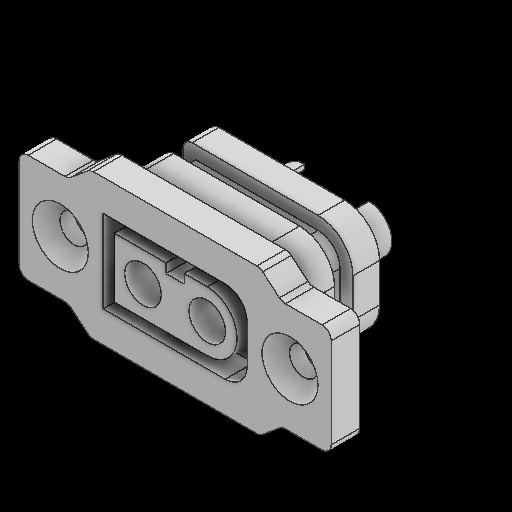
# Autodesk Inventor part: XT60E-F
Saved by Autodesk Inventor 2025.2 (Build 292293000, 293)
## iProperties
Created: 2026-06-05
Part Number: XT60E-F
Material: Generic
Document SubType Name: Modeling
Designer: valer
Density: 1 g/cm^3
Appearance: Default
Author: valer
Autodesk Inventor part; units mm, degrees
ref_plane "YZ Plane" through (0, 0, 0) normal (1, 0, 0) x (0, 1, 0)
ref_plane "XZ Plane" through (0, 0, 0) normal (0, 1, 0) x (-1, 0, 0)
ref_plane "XY Plane" through (0, 0, 0) normal (0, 0, 1) x (1, 0, 0)
sketch "Base" plane through (0, 0, 0) normal (0, 0, 1) x (1, 0, 0)
  line L0 (-17, 5.9) -> (17, 5.9)
  line L1 (17, 5.9) -> (17, -5.9)
  line L2 (17, -5.9) -> (-17, -5.9)
  line L3 (-17, -5.9) -> (-17, 5.9)
  line L4 (-17, 0) -> (17, 0) construction
  line L5 (-9.25, -7.9) -> (9.25, -7.9)
  line L6 (9.25, -7.9) -> (9.25, 7.9)
  line L7 (9.25, 7.9) -> (-9.25, 7.9)
  line L8 (-9.25, 7.9) -> (-9.25, -7.9)
  line L9 (-9.25, -7.9) -> (9.25, 7.9) construction
  line L10 (9.25, -7.9) -> (-9.25, 7.9) construction
  line L11 (-9.25, 7.9) -> (-11.6335, 5.9)
  line L12 (0, 7.9) -> (0, -7.9) construction
  line L13 (9.25, 7.9) -> (11.6335, 5.9)
  line L14 (-9.25, -7.9) -> (-11.6335, -5.9)
  line L15 (9.25, -7.9) -> (11.6335, -5.9)
  circle A0 centre (-12.5, 0) radius 1.55
  circle A1 centre (12.5, 0) radius 1.55
  arc A2 (9.25, 2.1) -> (5.45, 5.9) centre (5.45, 2.1) ccw
  arc A3 (5.45, -5.9) -> (9.25, -2.1) centre (5.45, -2.1) ccw
  circle A4 centre (3.5, 0) radius 2
  circle A5 centre (-3.5, 0) radius 2
  point P0 (0, 0)
  point P1 (0, 0)
  point P2 (0, 0)
  point P3 (5.45, -5.9)
  point P4 (9.25, -2.1)
  point P5 (-9.25, 5.9)
  point P6 (-9.25, -5.9)
  dimension "d0" = 11.8
  dimension "d1" = 15.8
  dimension "d2" = 18.5
  dimension "d3" = 140
  dimension "d4" = 3.1
  dimension "d5" = 3.8
  dimension "d6" = 4
  dimension "d7" = 3.5
  dimension "d8" = 25
  dimension "d9" = 34
  constraints: 32 end point, 8 midpoint, 8 symmetric about line, 6 centre point, 5 point on line, 4 parallel, 4 point on circle, 2 horizontal, 2 perpendicular, 2 tangent, 1 coincident, 3 other
  measures "d0" distance of L2.end L0.start
  measures "d1" distance of L7.end L5.start
  measures "d2" distance of L6.end L7.end
  measures "d3" angle of L7 L11
  measures "d4" diameter of A0
  measures "d5" radius of A2
  measures "d6" diameter of A4
  measures "d7" distance from line of A4.centre L12
  measures "d8" distance of A0.centre A1.centre
  measures "d9" distance between parallel lines of L1 L3
extrude "BaseFeature" add sketch "Base" along normal blind 3.1
fillet "BaseFilletsFeature" radius 1 12 edges at (-11.6335, -5.9, 1.55) (-17, -5.9, 1.55) (-9.25, -7.9, 1.55) (-17, 5.9, 1.55) (-11.6335, 5.9, 1.55) (-9.25, 7.9, 1.55) (9.25, -7.9, 1.55) (11.6335, -5.9, 1.55) (17, -5.9, 1.55) (17, 5.9, 1.55) (11.6335, 5.9, 1.55) (9.25, 7.9, 1.55)
extrude "BodyFeature" add sketch "Base" against normal blind 12.5 contours L0 A2 L6 A3 L2 L8
fillet "BodyFilletsFeature" radius 1 2 edges at (-9.25, -5.9, -6.25) (-9.25, 5.9, -6.25)
sketch "ReceptacleShroud" plane through (0, 0, 3.1) normal (0, 0, 1) x (1, 0, 0)
  line L0 (5.45, 5.9) -> (-8.25, 5.9) projected
  line L1 (-9.25, 4.9) -> (-9.25, -4.9) projected
  arc A0 (-8.25, 5.9) -> (-9.25, 4.9) centre (-8.25, 4.9) ccw projected
  arc A1 (9.25, 2.1) -> (5.45, 5.9) centre (5.45, 2.1) ccw projected
  line L2 (9.25, -2.1) -> (9.25, 2.1) projected
  arc A2 (5.45, -5.9) -> (9.25, -2.1) centre (5.45, -2.1) ccw projected
  line L3 (-8.25, -5.9) -> (5.45, -5.9) projected
  arc A3 (-9.25, -4.9) -> (-8.25, -5.9) centre (-8.25, -4.9) ccw projected
  line L4 (-7.85, 4.5) -> (5.45, 4.5)
  arc A4 (7.85, 2.1) -> (5.45, 4.5) centre (5.45, 2.1) ccw
  line L5 (7.85, 2.1) -> (7.85, -2.1)
  arc A5 (5.45, -4.5) -> (7.85, -2.1) centre (5.45, -2.1) ccw
  line L6 (5.45, -4.5) -> (-7.85, -4.5)
  line L7 (-7.85, -4.5) -> (-7.85, 4.5)
  line L8 (5.45, 3.25) -> (-6.6, 3.25) construction
  line L9 (-6.6, 3.25) -> (-6.6, -3.25)
  line L10 (-6.6, -3.25) -> (5.45, -3.25) construction
  arc A6 (5.45, -3.25) -> (6.6, -2.1) centre (5.45, -2.1) ccw construction
  line L11 (6.6, -2.1) -> (6.6, 2.1) construction
  arc A7 (6.6, 2.1) -> (5.45, 3.25) centre (5.45, 2.1) ccw construction
  line L12 (0, -11.06) -> (0, 11.06) construction
  line L13 (-1, 3.25) -> (-1, 2.25)
  line L14 (-1, 2.25) -> (1, 2.25)
  line L15 (1, 2.25) -> (1, 3.25)
  circle A8 centre (3.5, 0) radius 2 projected
  circle A9 centre (3.5, 0) radius 3.25
  line L16 (-6.6, 3.25) -> (3.5, 3.25)
  line L17 (-6.6, -3.25) -> (3.5, -3.25)
  point P0 (0, 0)
  point P1 (0, 2.25)
  dimension "d16" = 9
  dimension "d17" = 6.5
  dimension "d18" = 2
  dimension "d19" = 1
  constraints: 26 end point, 10 point on circle, 5 centre point, 5 point on line, 3 perpendicular, 1 coincident, 1 midpoint, 1 tangent, 10 other
  measures "d16" distance between parallel lines of L6 L4
  measures "d17" distance between parallel lines of L10 L8
  measures "d18" distance between parallel lines of L15 L13
  measures "d19" distance from line of L14.end L8
extrude "ReceptacleShroudFeature" cut sketch "ReceptacleShroud" against normal up to surface (3.1 mm away) contours L4 A4 L5 A5 L6 L7 | L16 L15 L14 L13
chamfer "MountHoleChamferFeature" distance 1.5 angle 45 2 edges at (-14.05, 0, 3.1) (10.95, 0, 3.1)
ref_plane "RidgePlane" through (0, 0, -7) normal (0, 0, -1) x (-1, 0, 0)
sketch "Ridge" plane through (0, 0, -7) normal (0, 0, -1) x (-1, 0, 0)
  arc A0 (9.25, 4.9) -> (8.25, 5.9) centre (8.25, 4.9) ccw projected
  line L0 (8.25, 5.9) -> (-5.45, 5.9) projected
  arc A1 (-5.45, 5.9) -> (-9.25, 2.1) centre (-5.45, 2.1) ccw projected
  line L1 (-9.25, 2.1) -> (-9.25, -2.1) projected
  arc A2 (-9.25, -2.1) -> (-5.45, -5.9) centre (-5.45, -2.1) ccw projected
  line L2 (-5.45, -5.9) -> (8.25, -5.9) projected
  arc A3 (8.25, -5.9) -> (9.25, -4.9) centre (8.25, -4.9) ccw projected
  line L3 (9.25, -4.9) -> (9.25, 4.9) projected
  circle A4 centre (3.5, 0) radius 2 projected
  circle A5 centre (-3.5, 0) radius 2 projected
  line L4 (7.85, -4.5) -> (-5.45, -4.5)
  arc A6 (-7.85, -2.1) -> (-5.45, -4.5) centre (-5.45, -2.1) ccw
  line L5 (-7.85, -2.1) -> (-7.85, 2.1)
  arc A7 (-5.45, 4.5) -> (-7.85, 2.1) centre (-5.45, 2.1) ccw
  line L6 (-5.45, 4.5) -> (7.85, 4.5)
  line L7 (7.85, 4.5) -> (7.85, -4.5)
  point P0 (0, 0)
  dimension "d26" = 15.7
  constraints: 8 end point, 4 point on circle, 2 centre point, 5 other
  measures "d26" distance between parallel lines of L5 L7
extrude "RidgeFeature" cut sketch "Ridge" against normal blind 2 contours L3 A3 L2 A2 L1 A1 L0 A0
split "BottomSculptFeature" plane through (0, 0, -9.9) removes the side toward (0, 0, -1)
ref_plane "BottomPlane" through (0, 0, -9.9) normal (0, 0, -1) x (-1, 0, 0)
sketch "Pins" plane through (5.45, -5.9, -9.9) normal (0, 0, -1) x (-1, 0, 0)
  circle A0 centre (8.95, 5.9) radius 2 projected
  circle A1 centre (1.95, 5.9) radius 2 projected
  circle A2 centre (1.95, 5.9) radius 2.5
  circle A3 centre (8.95, 5.9) radius 2.5
  point P0 (5.45, 5.9)
  dimension "d30" = 0.5
  dimension "d31" = 0.5
  constraints: 2 centre point
  measures "d30" radial gap between concentric circles of A1 A2
  measures "d31" radial gap between concentric circles of A0 A3
extrude "PinsFeature" add sketch "Pins" along normal blind 4.6
sketch "PinCuts" plane through (-8.25, -5.9, -7) normal (0, -1, 0) x (1, 0, 0)
  line L0 (2.25, -7.5) -> (7.25, -7.5) projected
  line L1 (9.25, -7.5) -> (14.25, -7.5) projected
  line L2 (2.25, -2.9) -> (2.25, -7.5) projected
  line L3 (14.25, -2.9) -> (14.25, -7.5) projected
  line L4 (4.75, -7.5) -> (11.75, -7.5)
  line L5 (11.75, -7.5) -> (11.75, -4.4)
  line L6 (11.75, -4.4) -> (4.75, -4.4)
  line L7 (4.75, -4.4) -> (4.75, -7.5)
  line L8 (13.7, -2.9) -> (0, -2.9) projected
  point P0 (8.25, 7)
  dimension "d34" = 1.5
  constraints: 8 end point, 2 midpoint, 2 parallel, 1 horizontal, 1 perpendicular
  measures "d34" distance between parallel lines of L6 L8
extrude "PinCutsFeature" cut sketch "PinCuts" against normal through all
body "Solid1"
